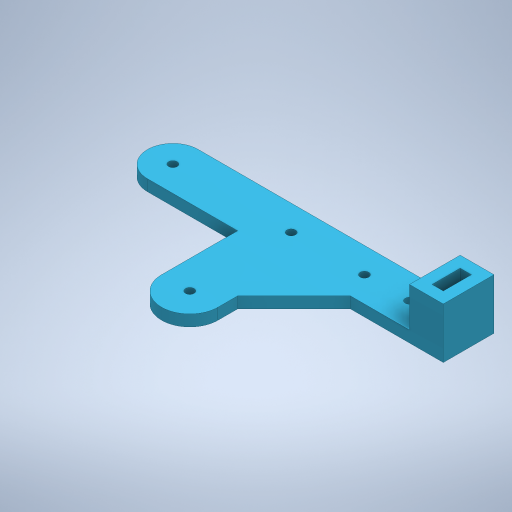
# Autodesk Inventor part: Fall-Wk-3 - Mounting Bracket 1of3
Saved by Autodesk Inventor 2024 (Build 280153000, 153)
## iProperties
Created: 2019-05-31
Part Number: Fall-Wk-3 - Mounting Bracket 1of3
Material: Generic
Document SubType Name: Modeling
Designer: cpmcdona
Density: 1 g/cm^3
Appearance: Turquoise
Author: cpmcdona
Autodesk Inventor part; units mm, degrees
ref_plane "YZ Plane" through (0, 0, 0) normal (1, 0, 0) x (0, 1, 0)
ref_plane "XZ Plane" through (0, 0, 0) normal (0, 1, 0) x (-1, 0, 0)
ref_plane "XY Plane" through (0, 0, 0) normal (0, 0, 1) x (1, 0, 0)
sketch "Sketch1" plane through (0, 0, 0) normal (0, 0, 1) x (1, 0, 0)
  line L0 (0, 0) -> (-100, 0)
  circle A0 centre (-100, -9) radius 1.5
  circle A1 centre (-16, -9) radius 1.5
  circle A2 centre (-58, -9) radius 1.5
  circle A3 centre (-58, -45) radius 1.5
  arc A4 (-100, 0) -> (-100, -18) centre (-100, -9) ccw
  arc A5 (-68, -45) -> (-48, -45) centre (-58, -45) ccw
  line L1 (0, -18) -> (-28, -18)
  line L2 (-28, -18) -> (-48, -38)
  line L3 (-48, -38) -> (-48, -45)
  line L4 (-68, -45) -> (-68, -18)
  line L5 (-68, -18) -> (-100, -18)
  line L6 (0, 0) -> (5, 0)
  line L7 (5, 0) -> (5, -18)
  line L8 (5, -18) -> (0, -18)
  dimension "d0" = 100
  dimension "d1" = 3
  dimension "d2" = 3
  dimension "d3" = 3
  dimension "d4" = 3
  dimension "d5" = 18
  dimension "d6" = 20
  dimension "d7" = 18
  dimension "d8" = 28
  dimension "d9" = 32
  dimension "d10" = 27
  dimension "d11" = 20
  dimension "d12" = 20
  dimension "d13" = 16
  dimension "d14" = 42
  dimension "d15" = 42
  dimension "d16" = 9
  dimension "d17" = 9
  dimension "d69" = 5
  dimension "d70" = 18
  dimension "d71" = 90
  constraints: 18 end point, 6 centre point, 4 point on circle, 2 coincident, 2 horizontal, 2 perpendicular, 2 point on line, 2 tangent, 1 parallel
  measures "d0" distance of L0.start L0.end
  measures "d1" diameter of A0
  measures "d2" diameter of A1
  measures "d3" diameter of A2
  measures "d4" diameter of A3
  measures "d5" diameter of A4
  measures "d6" diameter of A5
  measures "d7" distance of L0.start L1.start
  measures "d8" distance of L1.start L1.end
  measures "d9" distance of L4.end L5.end
  measures "d10" distance of L4.start L4.end
  measures "d11" horizontal distance of L1.end L2.end
  measures "d12" horizontal distance of L1.end L2.end
  measures "d13" horizontal distance of L0.start A1.centre
  measures "d14" distance of A2.centre A1.centre
  measures "d15" distance of A0.centre A2.centre
  measures "d16" distance from line of L0 A1.centre
  measures "d17" distance from line of L0 A2.centre
  measures "d69" distance of L0.start L6.end
  measures "d70" distance of L6.end L7.end
  measures "d71" angle of L6 L7
extrude "Extrusion7" add sketch "Sketch1" along normal blind 4
sketch "Sketch6" plane through (0, 0, 4) normal (0, 0, 1) x (1, 0, 0)
  line L0 (5, 0) -> (-100, 0) projected
  line L1 (5, 0) -> (-7, 0)
  line L2 (-7, 0) -> (-7, -18)
  line L3 (-7, -18) -> (5, -18)
  line L4 (5, -18) -> (5, 0)
  point P0 (0, 0)
  dimension "d74" = 12
  dimension "d75" = 18
  constraints: 8 end point, 2 parallel, 1 horizontal, 1 perpendicular
  measures "d74" distance of L3.end L2.end
  measures "d75" distance of L2.end L1.end
extrude "Extrusion8" add sketch "Sketch6" along normal blind 14
shell "Shell6" thickness 4 removed faces 1 at (-3, -12, 18)
sketch "Sketch7" plane through (0, 0, 4) normal (0, 0, 1) x (1, 0, 0)
  point P0 (0, 0)
sketch "Sketch8" plane through (0, 0, 4) normal (0, 0, 1) x (1, 0, 0)
  point P0 (0, 0)
sketch "Sketch9" plane through (0, 0, 4) normal (0, 0, 1) x (1, 0, 0)
  circle A0 centre (-32, -9) radius 1.5
  circle A1 centre (-16, -9) radius 1.5 projected
  line L0 (5, 0) -> (-7, 0) projected
  point P0 (0, 0)
  dimension "d79" = 3
  dimension "d80" = 16
  dimension "d81" = 9
  constraints: 1 centre point
  measures "d79" diameter of A0
  measures "d80" distance of A1.centre A0.centre
  measures "d81" distance from line of L0 A0.centre
extrude "Extrusion9" cut sketch "Sketch9" against normal through all contours A0
body "Solid2"
